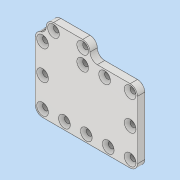
# Autodesk Inventor part: foreElectronicsSealingWallFrontCap
Saved by Autodesk Inventor 2017 (Build 210142000, 142)
## iProperties
Created: 2016-12-09
Part Number: foreElectronicsSealingWallFrontCap
Material: ABS Plastic
Document SubType Name: Modeling
Designer: techn
Density: 1.06 g/cm^3
Appearance: Smooth - White
Author: techn
Autodesk Inventor part; units mm, degrees
ref_plane "YZ Plane" through (0, 0, 0) normal (1, 0, 0) x (0, 1, 0)
ref_plane "XZ Plane" through (0, 0, 0) normal (0, 1, 0) x (-1, 0, 0)
ref_plane "XY Plane" through (0, 0, 0) normal (0, 0, 1) x (1, 0, 0)
sketch "Sketch4" plane through (0, 0, 0) normal (0, 0, 1) x (1, 0, 0)
  line L0 (15.875, 9.525) -> (15.875, -9.525)
  line L1 (15.875, -9.525) -> (-15.875, -9.525)
  line L2 (-15.875, -9.525) -> (-15.875, 9.525)
  line L3 (-15.875, 9.525) -> (-11.1125, 9.525)
  line L4 (-11.1125, 9.525) -> (-11.1125, 15.875)
  line L5 (-11.1125, 15.875) -> (-4.7625, 15.875)
  line L6 (-4.7625, 15.875) -> (-4.7625, 9.525)
  line L7 (-4.7625, 9.525) -> (15.875, 9.525)
  line L8 (1.5875, 22.225) -> (-17.4625, 22.225)
  line L9 (-17.4625, 22.225) -> (-17.4625, 15.875)
  line L10 (-17.4625, 15.875) -> (-22.225, 15.875)
  line L11 (-22.225, 15.875) -> (-22.225, -15.875)
  line L12 (-22.225, -15.875) -> (22.225, -15.875)
  line L13 (22.225, -15.875) -> (22.225, 15.875)
  line L14 (22.225, 15.875) -> (1.5875, 15.875)
  line L15 (1.5875, 15.875) -> (1.5875, 22.225)
  circle A0 centre (-14.2875, 19.05) radius 1.27
  circle A1 centre (-1.5875, 19.05) radius 1.27
  circle A2 centre (-1.5875, 12.7) radius 1.27
  circle A3 centre (7.9375, 12.7) radius 1.27
  circle A4 centre (19.05, 12.7) radius 1.27
  circle A5 centre (19.05, 0) radius 1.27
  circle A6 centre (19.05, -12.7) radius 1.27
  circle A7 centre (-19.05, 0) radius 1.27
  circle A8 centre (-19.05, -12.7) radius 1.27
  circle A9 centre (-9.525, -12.7) radius 1.27
  circle A10 centre (0, -12.7) radius 1.27
  circle A11 centre (9.525, -12.7) radius 1.27
  circle A12 centre (-19.05, 12.7) radius 1.27
  point P0 (0, 0)
  dimension "d95" = 2.54
  dimension "d96" = 2.54
  dimension "d97" = 2.54
  dimension "d98" = 2.54
  dimension "d99" = 2.54
  dimension "d100" = 2.54
  dimension "d101" = 2.54
  dimension "d102" = 2.54
  dimension "d103" = 2.54
  dimension "d104" = 2.54
  dimension "d105" = 2.54
  dimension "d106" = 2.54
  dimension "d107" = 3.175
  dimension "d108" = 3.175
  dimension "d109" = 3.175
  dimension "d110" = 3.175
  dimension "d111" = 3.175
  dimension "d112" = 3.175
  dimension "d113" = 9.525
  dimension "d114" = 9.525
  dimension "d115" = 9.525
  dimension "d116" = 9.525
  dimension "d117" = 2.54
  dimension "d118" = 3.175
  dimension "d119" = 3.175
  constraints: 32 end point, 13 centre point, 8 horizontal alignment, 4 vertical alignment
  measures "d95" diameter of A0
  measures "d96" diameter of A1
  measures "d97" diameter of A2
  measures "d98" diameter of A3
  measures "d99" diameter of A4
  measures "d100" diameter of A5
  measures "d101" diameter of A6
  measures "d102" diameter of A7
  measures "d103" diameter of A8
  measures "d104" diameter of A9
  measures "d105" diameter of A10
  measures "d106" diameter of A11
  measures "d107" distance from line of A0.centre L9
  measures "d108" distance from line of L8 A0.centre
  measures "d109" distance from line of L15 A2.centre
  measures "d110" distance from line of L11 A8.centre
  measures "d111" distance from line of L12 A8.centre
  measures "d112" distance from line of A4.centre L0
  measures "d113" distance of A3.centre A2.centre
  measures "d114" distance of A6.centre A11.centre
  measures "d115" distance of A10.centre A11.centre
  measures "d116" distance of A9.centre A10.centre
  measures "d117" diameter of A12
  measures "d118" distance from line of A12.centre L11
  measures "d119" distance from line of L10 A12.centre
extrude "Extrusion4" add sketch "Sketch4" along normal blind 3.175 contours L0 L1 L2 L3 L4 L5 L6 L7 | L15 L14 L13 L12 L11 L10 L9 L8
chamfer "Chamfer4" distance 1.27 angle 45 13 edges at (-15.5575, 19.05, 3.175) (-2.8575, 19.05, 3.175) (-2.8575, 12.7, 3.175) (6.6675, 12.7, 3.175) (17.78, 12.7, 3.175) (17.78, 0, 3.175) (17.78, -12.7, 3.175) (8.255, -12.7, 3.175) (-1.27, -12.7, 3.175) (-10.795, -12.7, 3.175) (-20.32, -12.7, 3.175) (-20.32, 0, 3.175) (-20.32, 12.7, 3.175)
fillet "Fillet3" radius 3.175 8 edges at (-17.4625, 22.225, 1.5875) (1.5875, 22.225, 1.5875) (1.5875, 15.875, 1.5875) (-17.4625, 15.875, 1.5875) (-22.225, 15.875, 1.5875) (22.225, 15.875, 1.5875) (22.225, -15.875, 1.5875) (-22.225, -15.875, 1.5875)
equation "\"d115\" = d114"
equation "\"d116\" = d114"
body "Solid4"
